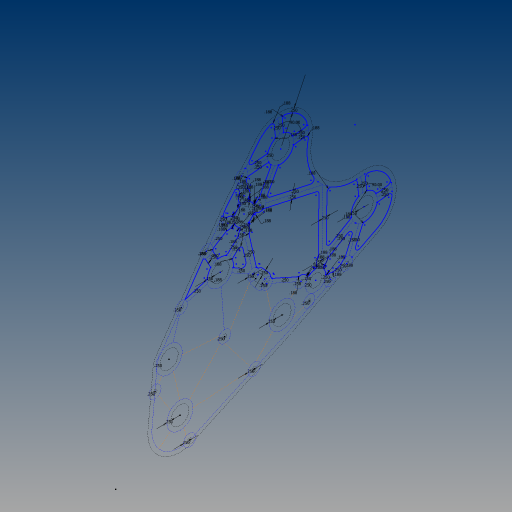
# Autodesk Inventor part: SHOT_1_001_ShooterPlate
Saved by Autodesk Inventor 2024.3 (Build 283343000, 343)
## iProperties
Created: 2024-08-07
Part Number: SHOT_1_001_ShooterPlate
Material: Aluminum 6061
Document SubType Name: Modeling
Designer: Kenji
Density: 2.7 g/cm^3
Appearance: Aluminum - Flat
Mass: 320.131 g
Surface Area: 825.953 cm^2
Volume: 118.567 cm^3
Author: Kenji
Autodesk Inventor part; units mm, degrees
ref_plane "YZ Plane" through (0, 0, 0) normal (1, 0, 0) x (0, 1, 0)
ref_plane "XZ Plane" through (0, 0, 0) normal (0, 1, 0) x (-1, 0, 0)
ref_plane "XY Plane" through (0, 0, 0) normal (0, 0, 1) x (1, 0, 0)
sketch "Sketch1" plane through (0, 0, 0) normal (1, 0, 0) x (0, 1, 0)
  line L0 (0, 0) -> (355.6, 0) construction
  line L1 (0, -355.6) -> (0, 0) construction
  line L2 (0, -292.1) -> (279.4, -292.1) construction
  circle A0 centre (336.7111, -261.0807) radius 50.8 construction
  circle A1 centre (191.0749, -393.5194) radius 50.8 construction
  circle A2 centre (263.893, -327.3) radius 50.8 construction
  circle A3 centre (191.0749, -393.5194) radius 47.625 construction
  circle A4 centre (336.7111, -261.0807) radius 47.625 construction
  line L3 (336.7111, -261.0807) -> (191.0749, -393.5194) construction
  circle A5 centre (336.7111, -261.0807) radius 14.2875
  circle A6 centre (191.0749, -393.5194) radius 14.2875
  circle A7 centre (215.3861, -165.4189) radius 25.4 construction
  circle A8 centre (107.6199, -263.4194) radius 25.4 construction
  circle A9 centre (107.6199, -263.4194) radius 22.225 construction
  circle A10 centre (215.3861, -165.4189) radius 22.225 construction
  circle A11 centre (215.3861, -165.4189) radius 14.2875
  circle A12 centre (107.6199, -263.4194) radius 14.2875
  line L4 (301.4765, -293.1223) -> (198.9433, -180.3717) construction
  line L5 (226.3095, -361.4778) -> (123.7762, -248.7272) construction
  circle A13 centre (161.3597, -214.5495) radius 50.8 construction
  line L6 (215.3861, -165.4189) -> (107.6199, -263.4194) construction
  circle A14 centre (50.8, -101.6) radius 50.8 construction
  circle A15 centre (25.4, -170.0653) radius 25.4 construction
  circle A16 centre (25.4, -170.0653) radius 22.225 construction
  circle A17 centre (25.4, -170.0653) radius 14.2875 construction
  circle A18 centre (136.3874, -84.4507) radius 25.4 construction
  circle A19 centre (136.3874, -84.4507) radius 22.225 construction
  circle A20 centre (136.3874, -84.4507) radius 14.2875
  circle A21 centre (50.8, -101.6) radius 14.2875
  circle A22 centre (41.2055, -25.7462) radius 25.4 construction
  circle A23 centre (41.2055, -25.7462) radius 22.225 construction
  circle A24 centre (41.2055, -25.7462) radius 14.2875 construction
  circle A25 centre (-111.1945, -98.7712) radius 50.8 construction
  circle A26 centre (41.2055, -98.7712) radius 50.8 construction
  line L7 (-111.1945, -47.9712) -> (41.2055, -47.9712) construction
  line L8 (-111.1945, -149.5712) -> (41.2055, -149.5712) construction
  circle A27 centre (276.2209, -203.0571) radius 30 construction
  circle A28 centre (276.2209, -203.0571) radius 25.4 construction
  circle A29 centre (301.6209, -203.0571) radius 2.794
  circle A30 centre (294.1814, -185.0966) radius 2.794
  circle A31 centre (276.2209, -177.6571) radius 2.794
  circle A32 centre (258.2604, -185.0966) radius 2.794
  circle A33 centre (250.8209, -203.0571) radius 2.794
  circle A34 centre (258.2604, -221.0177) radius 2.794
  circle A35 centre (276.2209, -228.4571) radius 2.794
  circle A36 centre (294.1814, -221.0177) radius 2.794
  circle A37 centre (276.2209, -203.0571) radius 9.652
  line L9 (250.7089, -187.273) -> (236.9862, -178.7828) construction
  circle A38 centre (276.2209, -203.0571) radius 9.5504 construction
  circle A39 centre (336.7111, -261.0807) radius 9.5504 construction
  circle A40 centre (336.7111, -261.0807) radius 14.3256 construction
  circle A41 centre (215.3861, -165.4189) radius 14.3256 construction
  circle A42 centre (136.3874, -84.4507) radius 14.3256 construction
  circle A43 centre (215.3861, -165.4189) radius 14.3256 construction
  circle A44 centre (123.5241, -172.549) radius 6.35 construction
  circle A45 centre (123.5241, -172.549) radius 3.2512
  line L10 (122.4294, -178.8039) -> (111.9989, -238.3998) construction
  arc A46 (325.875, -310.7115) -> (241.5089, -387.4324) centre (310.9542, -379.0508) ccw
  arc A47 (325.875, -310.7115) -> (368.3984, -221.3748) centre (336.7111, -261.0807) ccw
  arc A48 (145.82, -416.5983) -> (241.5089, -387.4324) centre (191.0749, -393.5194) ccw
  line L11 (138.8602, -59.1713) -> (55.7455, -51.0413)
  arc A49 (150.8617, -63.5783) -> (138.8602, -59.1713) centre (136.3874, -84.4507) ccw
  arc A50 (55.7455, -51.0413) -> (4.5541, -122.6227) centre (50.8, -101.6) ccw
  circle A51 centre (197.6195, -103.7307) radius 6.35 construction
  circle A52 centre (197.6195, -103.7307) radius 3.2512
  line L12 (161.503, -214.4192) -> (263.893, -327.3) construction
  circle A53 centre (128.5073, -316.6157) radius 30 construction
  circle A54 centre (128.5073, -316.6157) radius 25.4 construction
  circle A55 centre (152.1501, -307.3324) radius 2.794 construction
  line L13 (191.5627, -101.8236) -> (160.6148, -92.0791) construction
  line L14 (199.3769, -109.8327) -> (208.3565, -141.0111) construction
  line L15 (116.9032, -287.0622) -> (117.5428, -288.6911) construction
  circle A56 centre (128.5073, -316.6157) radius 22.86 construction
  circle A57 centre (107.6199, -263.4194) radius 34.29 construction
  circle A58 centre (138.661, -293.3334) radius 2.794
  circle A59 centre (119.224, -292.9729) radius 2.794 construction
  circle A60 centre (105.2251, -306.462) radius 2.794
  circle A61 centre (104.8646, -325.899) radius 2.794 construction
  circle A62 centre (118.3537, -339.8979) radius 2.794
  circle A63 centre (137.7907, -340.2584) radius 2.794 construction
  circle A64 centre (151.7896, -326.7693) radius 2.794
  line L16 (176.8412, -219.7225) -> (165.2897, -230.2004)
  line L17 (165.1271, -233.5371) -> (168.779, -237.5632)
  line L18 (172.1157, -237.7258) -> (183.6672, -227.2479)
  line L19 (183.8298, -223.9112) -> (180.1779, -219.8851)
  arc A65 (183.6672, -227.2479) -> (183.8298, -223.9112) centre (182.0802, -225.4982) ccw
  arc A66 (180.1779, -219.8851) -> (176.8412, -219.7225) centre (178.4283, -221.4722) ccw
  arc A67 (168.779, -237.5632) -> (172.1157, -237.7258) centre (170.5287, -235.9761) ccw
  arc A68 (165.2897, -230.2004) -> (165.1271, -233.5371) centre (166.8768, -231.9501) ccw
  line L20 (186.1428, -218.1439) -> (162.8049, -239.3128) construction
  circle A69 centre (186.1428, -218.1439) radius 2.3876
  circle A70 centre (162.8049, -239.3128) radius 2.3812
  circle A71 centre (128.5073, -316.6157) radius 9.5504
  circle A72 centre (276.2209, -203.0571) radius 30.48 construction
  circle A73 centre (336.7111, -261.0807) radius 41.91 construction
  circle A74 centre (276.2209, -203.0571) radius 41.91 construction
  circle A75 centre (128.5073, -316.6157) radius 19.1008 construction
  circle A76 centre (215.3861, -165.4189) radius 19.1008 construction
  circle A77 centre (136.3874, -84.4507) radius 19.1008 construction
  circle A78 centre (276.2209, -203.0571) radius 19.1008 construction
  circle A79 centre (191.0749, -393.5194) radius 19.1008 construction
  line L21 (4.5541, -122.6227) -> (75.2478, -278.1353)
  line L22 (75.9415, -279.5746) -> (145.82, -416.5983)
  arc A80 (75.2478, -278.1353) -> (75.9415, -279.5746) centre (107.6199, -263.4194) ccw
  circle A81 centre (276.2209, -203.0571) radius 43.18 construction
  line L23 (303.1551, -169.3072) -> (368.3984, -221.3748)
  line L24 (150.8617, -63.5783) -> (300.8271, -167.5741)
  arc A82 (303.1551, -169.3072) -> (300.8271, -167.5741) centre (276.2209, -203.0571) ccw
  circle A83 centre (107.6199, -263.4194) radius 35.56 construction
  circle A84 centre (126.9785, -365.675) radius 6.35 construction
  circle A85 centre (126.9785, -365.675) radius 3.2512
  circle A86 centre (330.5575, -199.3) radius 6.35 construction
  circle A87 centre (330.5575, -199.3) radius 3.2512
  circle A88 centre (255.1053, -143.5951) radius 6.35
  circle A89 centre (255.1053, -143.5951) radius 3.2512
  circle A90 centre (103.0707, -62.0508) radius 6.35 construction
  circle A91 centre (103.0707, -62.0508) radius 3.2512
  circle A92 centre (9.0853, -116.952) radius 6.35 construction
  circle A93 centre (9.0853, -116.952) radius 3.2512
  line L25 (37.3917, -106.5346) -> (15.0445, -114.7588) construction
  line L26 (10.9498, -123.0221) -> (17.9418, -145.7849) construction
  line L27 (108.3404, -65.5938) -> (115.3086, -70.2787) construction
  line L28 (98.0069, -65.8823) -> (91.3109, -70.9486) construction
  line L29 (257.2302, -149.579) -> (261.7713, -162.3666) construction
  line L30 (249.54, -146.6529) -> (237.6471, -153.1876) construction
  line L31 (331.1869, -205.6187) -> (331.6761, -210.5308) construction
  line L32 (324.2226, -199.738) -> (319.298, -200.0785) construction
  line L33 (127.1763, -359.3281) -> (127.5729, -346.6011) construction
  line L34 (132.8027, -368.2051) -> (144.4815, -373.2786) construction
  line L35 (38.6307, -191.7472) -> (52.2676, -214.0948) construction
  line L36 (80.4395, -240.4904) -> (60.4289, -223.6098) construction
  circle A94 centre (55.5753, -219.5153) radius 6.35 construction
  circle A95 centre (55.5753, -219.5153) radius 3.2512
  point P0 (33.8339, -53.7169)
  point P1 (178.5909, -218.1355)
  point P2 (163.5401, -231.7874)
  point P3 (170.3661, -239.3128)
  point P4 (171.0655, -224.9615)
  point P5 (182.0039, -221.8982)
  point P6 (182.0039, -221.8982)
  dimension "d44" = 101.6
  dimension "d60" = 28.575
  dimension "d81" = 60
  dimension "d82" = 50.8
  dimension "d102" = 12.7
  dimension "d269" = 50.8
  dimension "d13" = 355.6
  dimension "d14" = 355.6
  dimension "d15" = 292.1
  dimension "d29" = 101.6
  dimension "d31" = 3.175
  dimension "d36" = 28.575
  dimension "d38" = 50.8
  dimension "d39" = 3.175
  dimension "d41" = 28.575
  dimension "d42" = 152.4
  dimension "d43" = 152.4
  dimension "d46" = 279.4
  dimension "d47" = 101.6
  dimension "d50" = 101.6
  dimension "d51" = 145.6628
  dimension "d61" = 113.1223
  dimension "d77" = 101.6
  dimension "d78" = 101.6
  dimension "d79" = 152.4
  dimension "d80" = 41.2055
  dimension "d83" = 5.588
  dimension "d86" = 360
  dimension "d88" = 19.304
  dimension "d91" = 19.1008
  dimension "d92" = 19.1008
  dimension "d93" = 28.6512
  dimension "d94" = 28.6512
  dimension "d95" = 28.6512
  dimension "d96" = 28.6512
  dimension "d103" = 6.5024
  dimension "d108" = 12.7
  dimension "d109" = 6.5024
  dimension "d114" = 101.6
  dimension "d116" = 87.2886
  dimension "d117" = 158.0611
  dimension "d119" = 323.8734
  dimension "d121" = 42.21
  dimension "d268" = 60
  dimension "d270" = 5.588
  dimension "d279" = 45.72
  dimension "d280" = 68.58
  dimension "d283" = 360
  dimension "d285" = 20.32
  dimension "d286" = 10.16
  dimension "d287" = 10.16
  dimension "d288" = 2.3622
  dimension "d289" = 2.3622
  dimension "d291" = 5.08
  dimension "d292" = 4.7752
  dimension "d293" = 4.7625
  dimension "d294" = 5.6005
  dimension "d295" = 5.588
  dimension "d296" = 19.1008
  dimension "d297" = 60.96
  dimension "d300" = 83.82
  dimension "d301" = 83.82
  dimension "d302" = 38.2016
  dimension "d303" = 38.2016
  dimension "d304" = 38.2016
  dimension "d305" = 38.2016
  dimension "d306" = 38.2016
  dimension "d309" = 1.27
  dimension "d312" = 1.27
  dimension "d314" = 208.6282
  constraints: 89 centre point, 74 end point, 71 point on circle, 46 point on line, 46 tangent, 38 coincident, 18 equal radius, 7 equal length, 6 concentric, 6 midpoint, 5 perpendicular, 3 horizontal, 2 horizontal alignment, 2 parallel, 1 vertical alignment, 60 other
  measures "d13" distance of L1.start L0.start
  measures "d14" distance of L0.start L0.end
  measures "d15" distance between parallel lines of L0 L2
  measures "d29" diameter of A1
  measures "d31" radial gap between concentric circles of A1 A3
  measures "d36" diameter of A5
  measures "d38" diameter of A8
  measures "d39" radial gap between concentric circles of A8 A9
  measures "d41" diameter of A12
  measures "d42" distance of L4.start L4.end
  measures "d43" distance of L5.start L5.end
  measures "d46" distance of L2.start L2.end
  measures "d47" diameter of A14
  measures "d50" distance from line of L0 A14.centre
  measures "d51" distance of L6.start L6.end
  measures "d61" distance of A19.centre A7.centre
  measures "d77" diameter of A25
  measures "d78" diameter of A26
  measures "d79" distance of L8.start L8.end
  measures "d80" distance from line of L1 A22.centre
  measures "d83" diameter of A29
  measures "d88" diameter of A37
  measures "d91" diameter of A38
  measures "d92" diameter of A39
  measures "d93" diameter of A40
  measures "d94" diameter of A41
  measures "d95" diameter of A42
  measures "d96" diameter of A43
  measures "d103" diameter of A45
  measures "d108" diameter of A51
  measures "d109" diameter of A52
  measures "d114" distance of point (123.524, -172.549) A14.centre
  measures "d116" distance of A14.centre A19.centre
  measures "d117" distance of A14.centre L12.start
  measures "d119" distance of A14.centre L3.end
  measures "d121" angle of L1 L12
  measures "d268" diameter of A53
  measures "d270" diameter of A55
  measures "d279" diameter of A56
  measures "d280" diameter of A57
  measures "d285" distance of point (178.591, -218.135) point (163.54, -231.787)
  measures "d286" distance of point (163.54, -231.787) point (170.366, -239.313)
  measures "d287" distance of point (178.591, -218.135) point (171.065, -224.961)
  measures "d288" radius of A65
  measures "d289" radius of A67
  measures "d291" distance between parallel lines of L16 L20
  measures "d292" diameter of A69
  measures "d293" diameter of A70
  measures "d294" distance from line of L17 L20.end
  measures "d295" distance from line of L19 A69.centre
  measures "d296" diameter of A71
  measures "d297" diameter of A72
  measures "d300" diameter of A73
  measures "d301" diameter of A74
  measures "d302" diameter of A75
  measures "d303" diameter of A76
  measures "d304" diameter of A77
  measures "d305" diameter of A78
  measures "d306" diameter of A79
  measures "d309" radial gap between concentric circles of A74 A81
  measures "d312" radial gap between concentric circles of A57 A83
  measures "d314" distance of L3.end point (276.221, -203.057)
extrude "Extrusion6" add sketch "Sketch1" along normal blind 4.7625 contours A30 | A32 | A34 | A36 | A88 | A46 A48 L22 A80 L21 A50 L11 A49 L24 A82 L23 A47 | A85 | A87 | A89 | A91 | A93 | A95
extrude "Extrusion7" cut sketch "Sketch1" along normal blind 25.4 contours A85 | A87 | A89 | A91 | A93 | A95
sketch "Sketch5" plane through (4.7625, 0, 0) normal (1, 0, 0) x (0, 0, -1)
  circle A0 centre (62.0508, 103.0707) radius 3.2512 construction
  circle A1 centre (365.675, 126.9785) radius 3.2512 construction
  circle A2 centre (116.952, 9.0853) radius 3.2512 construction
  circle A3 centre (143.5951, 255.1053) radius 3.2512 construction
  circle A4 centre (199.3, 330.5575) radius 3.2512 construction
  circle A5 centre (219.5153, 55.5753) radius 3.2512 construction
  line L0 (167.5741, 300.8271) -> (63.5783, 150.8617) construction
  arc A6 (63.5783, 150.8617) -> (59.1713, 138.8602) centre (84.4507, 136.3874) ccw construction
  line L1 (59.1713, 138.8602) -> (51.0413, 55.7455) construction
  arc A7 (51.0413, 55.7455) -> (122.6227, 4.5541) centre (101.6, 50.8) ccw construction
  line L2 (122.6227, 4.5541) -> (278.1353, 75.2478) construction
  arc A8 (278.1353, 75.2478) -> (279.5746, 75.9415) centre (263.4194, 107.6199) ccw construction
  line L3 (279.5746, 75.9415) -> (416.5983, 145.82) construction
  arc A9 (416.5983, 145.82) -> (387.4324, 241.5089) centre (393.5194, 191.0749) ccw construction
  arc A10 (310.7115, 325.875) -> (387.4324, 241.5089) centre (379.0508, 310.9542) ccw construction
  arc A11 (310.7115, 325.875) -> (221.3748, 368.3984) centre (261.0807, 336.7111) ccw construction
  line L4 (221.3748, 368.3984) -> (169.3072, 303.1551) construction
  arc A12 (169.3072, 303.1551) -> (167.5741, 300.8271) centre (203.0571, 276.2209) ccw construction
  circle A13 centre (326.7693, 151.7896) radius 2.794 construction
  circle A14 centre (172.549, 123.5241) radius 3.2512 construction
  circle A15 centre (203.0571, 276.2209) radius 9.652 construction
  circle A16 centre (228.4571, 276.2209) radius 2.794 construction
  circle A17 centre (203.0571, 250.8209) radius 2.794 construction
  circle A18 centre (177.6571, 276.2209) radius 2.794 construction
  circle A19 centre (84.4507, 136.3874) radius 14.2875 construction
  circle A20 centre (263.4194, 107.6199) radius 14.2875 construction
  circle A21 centre (316.6157, 128.5073) radius 9.5504 construction
  circle A22 centre (239.3128, 162.8049) radius 2.3812 construction
  circle A23 centre (218.1439, 186.1428) radius 2.3876 construction
  arc A24 (219.8851, 180.1779) -> (219.7225, 176.8412) centre (221.4722, 178.4283) ccw construction
  line L5 (219.8851, 180.1779) -> (223.9112, 183.8298) construction
  arc A25 (227.2479, 183.6672) -> (223.9112, 183.8298) centre (225.4982, 182.0802) ccw construction
  line L6 (227.2479, 183.6672) -> (237.7258, 172.1157) construction
  arc A26 (237.5632, 168.779) -> (237.7258, 172.1157) centre (235.9761, 170.5287) ccw construction
  line L7 (237.5632, 168.779) -> (233.5371, 165.1271) construction
  arc A27 (230.2004, 165.2897) -> (233.5371, 165.1271) centre (231.9501, 166.8768) ccw construction
  line L8 (230.2004, 165.2897) -> (219.7225, 176.8412) construction
  circle A28 centre (339.8979, 118.3537) radius 2.794 construction
  circle A29 centre (306.462, 105.2251) radius 2.794 construction
  circle A30 centre (293.3334, 138.661) radius 2.794 construction
  circle A31 centre (103.7307, 197.6195) radius 3.2512 construction
  circle A32 centre (203.0571, 301.6209) radius 2.794 construction
  circle A33 centre (101.6, 50.8) radius 14.2875 construction
  circle A34 centre (165.4189, 215.3861) radius 14.2875 construction
  circle A35 centre (393.5194, 191.0749) radius 14.2875 construction
  circle A36 centre (261.0807, 336.7111) radius 14.2875 construction
  arc A37 (304.5076, 327.2295) -> (226.3381, 364.4375) centre (261.0807, 336.7111) ccw construction
  arc A38 (304.5076, 327.2295) -> (388.1933, 235.2047) centre (379.0508, 310.9542) ccw construction
  arc A39 (413.7134, 151.4769) -> (388.1933, 235.2047) centre (393.5194, 191.0749) ccw construction
  line L9 (413.7134, 151.4769) -> (276.6898, 81.5983) construction
  arc A40 (275.5075, 81.0285) -> (276.6898, 81.5983) centre (263.4194, 107.6199) ccw construction
  line L10 (275.5075, 81.0285) -> (119.9949, 10.3348) construction
  arc A41 (57.3611, 55.1273) -> (119.9949, 10.3348) centre (101.6, 50.8) ccw construction
  line L11 (57.3611, 55.1273) -> (65.4912, 138.242) construction
  arc A42 (68.7964, 147.2431) -> (65.4912, 138.242) centre (84.4507, 136.3874) ccw construction
  line L12 (68.7964, 147.2431) -> (172.7922, 297.2086) construction
  arc A43 (174.2704, 299.1942) -> (172.7922, 297.2086) centre (203.0571, 276.2209) ccw construction
  line L13 (174.2704, 299.1942) -> (226.3381, 364.4375) construction
  circle A44 centre (261.0807, 336.7111) radius 20.6375 construction
  circle A45 centre (199.3, 330.5575) radius 9.6012 construction
  circle A46 centre (203.0571, 301.6209) radius 9.144 construction
  circle A47 centre (228.4571, 276.2209) radius 9.144 construction
  circle A48 centre (203.0571, 276.2209) radius 16.002 construction
  circle A49 centre (177.6571, 276.2209) radius 9.144 construction
  circle A50 centre (203.0571, 250.8209) radius 9.144 construction
  circle A51 centre (143.5951, 255.1053) radius 9.6012 construction
  circle A52 centre (165.4189, 215.3861) radius 20.6375 construction
  circle A53 centre (103.7307, 197.6195) radius 9.6012 construction
  circle A54 centre (84.4507, 136.3874) radius 20.6375 construction
  circle A55 centre (62.0508, 103.0707) radius 9.6012 construction
  circle A56 centre (172.549, 123.5241) radius 9.6012 construction
  circle A57 centre (101.6, 50.8) radius 20.6375 construction
  circle A58 centre (116.952, 9.0853) radius 9.6012 construction
  circle A59 centre (219.5153, 55.5753) radius 9.6012 construction
  circle A60 centre (263.4194, 107.6199) radius 20.6375 construction
  circle A61 centre (218.1439, 186.1428) radius 8.7376 construction
  line L14 (242.4292, 176.382) -> (231.9513, 187.9335) construction
  arc A62 (231.9513, 187.9335) -> (219.6449, 188.5332) centre (225.4982, 182.0802) ccw construction
  line L15 (219.6449, 188.5332) -> (215.6189, 184.8813) construction
  arc A63 (215.6189, 184.8813) -> (215.0191, 172.575) centre (221.4722, 178.4283) ccw construction
  line L16 (215.0191, 172.575) -> (225.497, 161.0235) construction
  arc A64 (225.497, 161.0235) -> (237.8033, 160.4238) centre (231.9501, 166.8768) ccw construction
  line L17 (237.8033, 160.4238) -> (241.8294, 164.0757) construction
  arc A65 (241.8294, 164.0757) -> (242.4292, 176.382) centre (235.9761, 170.5287) ccw construction
  circle A66 centre (239.3128, 162.8049) radius 8.7312 construction
  circle A67 centre (393.5194, 191.0749) radius 20.6375 construction
  circle A68 centre (326.7693, 151.7896) radius 9.144 construction
  circle A69 centre (293.3334, 138.661) radius 9.144 construction
  circle A70 centre (316.6157, 128.5073) radius 15.9004 construction
  circle A71 centre (365.675, 126.9785) radius 9.6012 construction
  circle A72 centre (339.8979, 118.3537) radius 9.144 construction
  circle A73 centre (306.462, 105.2251) radius 9.144 construction
  line L18 (240.5448, 334.6656) -> (208.8539, 331.5091) construction
  line L19 (259.0352, 357.247) -> (256.6751, 380.9422) construction
  line L20 (281.6165, 338.7565) -> (305.3118, 341.1167) construction
  line L21 (251.2843, 318.5469) -> (232.7977, 284.269) construction
  line L22 (200.5362, 321.0362) -> (201.8798, 310.6888) construction
  line L23 (170.1431, 281.4316) -> (164.544, 285.3144) construction
  line L24 (148.2185, 246.6906) -> (155.4809, 233.4731) construction
  line L25 (151.7555, 260.1641) -> (169.8853, 271.403) construction
  line L26 (205.0841, 241.9044) -> (215.844, 194.5723) construction
  line L27 (183.5074, 205.4507) -> (210.6081, 190.5652) construction
  line L28 (180.4451, 229.5325) -> (196.3994, 244.5529) construction
  line L29 (252.4974, 358.8173) -> (250.9874, 373.9773)
  line L30 (237.7157, 340.7653) -> (216.1032, 338.6126)
  line L31 (211.8976, 346.3429) -> (226.3381, 364.4375)
  arc A74 (244.449, 377.9323) -> (226.3381, 364.4375) centre (261.0807, 336.7111) ccw
  arc A75 (250.2514, 354.2791) -> (241.7218, 343.8623) centre (261.0807, 336.7111) ccw
  arc A76 (250.2514, 354.2791) -> (252.4974, 358.8173) centre (247.7457, 358.344) ccw
  arc A77 (237.7157, 340.7653) -> (241.7218, 343.8623) centre (237.2424, 345.5169) ccw
  arc A78 (211.8976, 346.3429) -> (216.1032, 338.6126) centre (215.6299, 343.3643) ccw
  arc A79 (250.9874, 373.9773) -> (244.449, 377.9323) centre (246.2357, 373.504) ccw
  line L32 (238.9744, 328.1278) -> (211.3352, 325.3748)
  line L33 (207.073, 320.0083) -> (208.2772, 310.7339)
  line L34 (244.646, 319.6154) -> (226.8389, 286.5977)
  arc A80 (206.5244, 324.2336) -> (207.0953, 324.9525) centre (199.3, 330.5575) ccw
  arc A81 (243.5127, 325.8818) -> (244.321, 324.6686) centre (261.0807, 336.7111) ccw
  line L35 (219.0591, 276.2209) -> (219.3131, 276.2209) construction
  line L36 (203.0571, 292.4769) -> (203.0571, 292.2229) construction
  line L37 (209.4071, 294.0954) -> (209.4071, 292.4021)
  line L38 (219.2384, 282.5709) -> (220.9317, 282.5709)
  arc A82 (209.9856, 295.6536) -> (209.5973, 308.0115) centre (203.0571, 301.6209) ccw
  arc A83 (217.1375, 283.824) -> (210.6603, 290.3012) centre (203.0571, 276.2209) ccw
  arc A84 (224.633, 284.5268) -> (222.4898, 283.1494) centre (228.4571, 276.2209) ccw
  arc A85 (211.3352, 325.3748) -> (207.073, 320.0083) centre (211.8085, 320.6231) ccw
  arc A86 (243.5127, 325.8818) -> (238.9744, 328.1278) centre (239.4477, 323.3761) ccw
  arc A87 (244.646, 319.6154) -> (244.321, 324.6686) centre (240.4431, 321.8822) ccw
  arc A88 (224.633, 284.5268) -> (226.8389, 286.5977) centre (222.636, 288.8644) ccw
  arc A89 (208.2772, 310.7339) -> (209.5973, 308.0115) centre (213.0127, 311.3488) ccw
  circle A90 centre (211.7947, 294.0954) radius 2.3876 construction
  circle A91 centre (220.9317, 284.9585) radius 2.3876 construction
  circle A92 centre (219.2384, 284.9585) radius 2.3876 construction
  circle A93 centre (211.7947, 292.4021) radius 2.3876 construction
  arc A94 (217.1375, 283.824) -> (219.2384, 282.5709) centre (219.2384, 284.9585) ccw
  arc A95 (220.9317, 282.5709) -> (222.4898, 283.1494) centre (220.9317, 284.9585) ccw
  arc A96 (209.4071, 292.4021) -> (210.6603, 290.3012) centre (211.7947, 292.4021) ccw
  arc A97 (209.9856, 295.6536) -> (209.4071, 294.0954) centre (211.7947, 294.0954) ccw
  line L39 (328.2576, 254.0189) -> (237.3829, 274.2352) construction
  line L40 (328.2576, 254.0189) -> (326.9024, 160.9326) construction
  line L41 (255.824, 313.5869) -> (241.0284, 286.1531)
  line L42 (244.1944, 279.2252) -> (308.259, 264.9731)
  line L43 (284.4456, 332.6569) -> (299.6056, 334.1669)
  arc A98 (260.2249, 316.0913) -> (280.4395, 329.5599) centre (261.0807, 336.7111) ccw
  arc A99 (304.5076, 327.2295) -> (304.7726, 328.5371) centre (261.0807, 336.7111) ccw
  arc A100 (304.5076, 327.2295) -> (313.4045, 272.0681) centre (379.0508, 310.9542) ccw
  arc A101 (304.7726, 328.5371) -> (299.6056, 334.1669) centre (300.0789, 329.4152) ccw
  arc A102 (308.259, 264.9731) -> (313.4045, 272.0681) centre (309.296, 269.6344) ccw
  arc A103 (241.0284, 286.1531) -> (244.1944, 279.2252) centre (245.2313, 283.8864) ccw
  arc A104 (260.2249, 316.0913) -> (255.824, 313.5869) centre (260.0269, 311.3202) ccw
  arc A105 (284.4456, 332.6569) -> (280.4395, 329.5599) centre (284.9189, 327.9052) ccw
  line L44 (283.1869, 345.2944) -> (298.3468, 346.8044)
  line L45 (265.1348, 360.076) -> (263.6248, 375.236)
  arc A106 (302.3019, 353.3428) -> (269.2547, 380.403) centre (261.0807, 336.7111) ccw
  arc A107 (278.6486, 347.5403) -> (268.2318, 356.07) centre (261.0807, 336.7111) ccw
  arc A108 (269.2547, 380.403) -> (263.6248, 375.236) centre (268.3765, 375.7093) ccw
  arc A109 (298.3468, 346.8044) -> (302.3019, 353.3428) centre (297.8735, 351.556) ccw
  arc A110 (278.6486, 347.5403) -> (283.1869, 345.2944) centre (282.7136, 350.046) ccw
  arc A111 (265.1348, 360.076) -> (268.2318, 356.07) centre (269.8865, 360.5493) ccw
  line L46 (235.2436, 268.2059) -> (318.0387, 249.787)
  line L47 (321.7764, 245.0563) -> (320.5418, 160.2462)
  line L48 (211.1035, 244.0716) -> (222.1565, 195.4498)
  line L49 (203.0571, 260.2189) -> (203.0571, 259.9649) construction
  line L50 (209.4071, 260.0397) -> (209.4071, 258.3463)
  line L51 (247.2842, 159.2422) -> (284.9853, 142.3921) construction
  line L52 (248.8959, 165.4772) -> (288.2875, 147.8716)
  line L53 (301.715, 135.0057) -> (302.041, 134.8635) construction
  line L54 (323.114, 143.408) -> (322.9719, 143.082) construction
  line L55 (302.7698, 141.4733) -> (304.4279, 140.7502)
  line L56 (317.6048, 146.6604) -> (317.2174, 145.7719)
  arc A112 (301.5729, 142.6264) -> (291.2986, 147.5757) centre (293.3334, 138.661) ccw
  arc A113 (319.5416, 157.3907) -> (317.8734, 149.6741) centre (326.7693, 151.7896) ccw
  arc A114 (315.236, 144.3478) -> (306.8489, 141.0546) centre (316.6157, 128.5073) ccw
  line L57 (219.2384, 269.8709) -> (220.9317, 269.8709)
  arc A115 (222.4898, 269.2924) -> (232.2342, 267.8934) centre (228.4571, 276.2209) ccw
  arc A116 (210.6603, 262.1405) -> (217.1375, 268.6177) centre (203.0571, 276.2209) ccw
  arc A117 (211.402, 247.0824) -> (209.9856, 256.7882) centre (203.0571, 250.8209) ccw
  arc A118 (235.2436, 268.2059) -> (232.2342, 267.8934) centre (234.2067, 263.5446) ccw
  arc A119 (321.7764, 245.0563) -> (318.0387, 249.787) centre (317.0017, 245.1258) ccw
  arc A120 (319.5416, 157.3907) -> (320.5418, 160.2462) centre (315.7671, 160.3157) ccw
  arc A121 (317.6048, 146.6604) -> (317.8734, 149.6741) centre (313.2278, 148.5693) ccw
  arc A122 (224.5561, 192.0782) -> (223.7494, 192.8453) centre (218.1439, 186.1428) ccw
  arc A123 (231.9513, 187.9335) -> (227.1533, 190.6337) centre (225.4982, 182.0802) ccw
  arc A124 (246.7674, 167.3507) -> (245.8371, 168.6073) centre (239.3128, 162.8049) ccw
  arc A125 (244.6507, 171.3375) -> (242.4292, 176.382) centre (235.9761, 170.5287) ccw
  line L58 (231.9513, 187.9335) -> (242.4292, 176.382)
  arc A126 (211.402, 247.0824) -> (211.1035, 244.0716) centre (215.7599, 245.1301) ccw
  arc A127 (222.1565, 195.4498) -> (223.7494, 192.8453) centre (226.8129, 196.5083) ccw
  arc A128 (224.5561, 192.0782) -> (227.1533, 190.6337) centre (228.0605, 195.3219) ccw
  arc A129 (244.6507, 171.3375) -> (245.8371, 168.6073) centre (249.4053, 171.7808) ccw
  arc A130 (246.7674, 167.3507) -> (248.8959, 165.4772) centre (250.8444, 169.8368) ccw
  arc A131 (288.2875, 147.8716) -> (291.2986, 147.5757) centre (290.2359, 152.2312) ccw
  circle A132 centre (211.7947, 258.3463) radius 2.3876 construction
  circle A133 centre (211.7947, 260.0397) radius 2.3876 construction
  circle A134 centre (220.9317, 267.4833) radius 2.3876 construction
  circle A135 centre (219.2384, 267.4833) radius 2.3876 construction
  arc A136 (219.2384, 269.8709) -> (217.1375, 268.6177) centre (219.2384, 267.4833) ccw
  arc A137 (222.4898, 269.2924) -> (220.9317, 269.8709) centre (220.9317, 267.4833) ccw
  arc A138 (210.6603, 262.1405) -> (209.4071, 260.0397) centre (211.7947, 260.0397) ccw
  arc A139 (209.4071, 258.3463) -> (209.9856, 256.7882) centre (211.7947, 258.3463) ccw
  circle A140 centre (315.0288, 146.7264) radius 2.3876 construction
  circle A141 centre (303.7243, 143.6618) radius 2.3876 construction
  circle A142 centre (305.3824, 142.9387) radius 2.3876 construction
  arc A143 (315.236, 144.3478) -> (317.2174, 145.7719) centre (315.0288, 146.7264) ccw
  arc A144 (301.5729, 142.6264) -> (302.7698, 141.4733) centre (303.7243, 143.6618) ccw
  arc A145 (304.4279, 140.7502) -> (306.8489, 141.0546) centre (305.3824, 142.9387) ccw
  line L59 (385.2966, 172.1463) -> (369.5005, 135.7847) construction
  line L60 (375.7337, 180.6072) -> (334.6498, 156.4276) construction
  line L61 (391.0466, 211.5637) -> (388.1933, 235.2047) construction
  line L62 (414.0082, 193.5478) -> (437.6492, 196.4011) construction
  line L63 (333.4067, 171.4846) -> (334.4104, 240.4277)
  line L64 (370.6077, 184.9585) -> (340.6035, 167.2997)
  line L65 (384.4774, 212.9975) -> (382.3693, 230.4644)
  arc A146 (382.3265, 208.4134) -> (372.946, 189.4499) centre (393.5194, 191.0749) ccw
  arc A147 (341.5331, 244.5162) -> (377.7123, 234.6667) centre (379.0508, 310.9542) ccw
  arc A148 (341.5331, 244.5162) -> (334.4104, 240.4277) centre (339.1851, 240.3582) ccw
  arc A149 (382.3693, 230.4644) -> (377.7123, 234.6667) centre (377.6285, 229.8922) ccw
  arc A150 (382.3265, 208.4134) -> (384.4774, 212.9975) centre (379.7366, 212.4253) ccw
  arc A151 (370.6077, 184.9585) -> (372.946, 189.4499) centre (368.1856, 189.0739) ccw
  arc A152 (333.4067, 171.4846) -> (340.6035, 167.2997) centre (338.1814, 171.4151) ccw
  line L66 (367.2672, 168.2562) -> (337.1993, 150.5599)
  line L67 (374.069, 162.2382) -> (363.4789, 137.8602)
  line L68 (348.5694, 121.2551) -> (356.57, 123.932) construction
  line L69 (345.8158, 127.0298) -> (355.0252, 130.1112)
  arc A153 (361.2833, 135.5164) -> (357.5507, 132.0949) centre (365.675, 126.9785) ccw
  arc A154 (355.0252, 130.1112) -> (357.5507, 132.0949) centre (353.51, 134.6396) ccw
  arc A155 (361.2833, 135.5164) -> (363.4789, 137.8602) centre (359.0991, 139.7628) ccw
  arc A156 (374.069, 162.2382) -> (367.2672, 168.2562) centre (369.6893, 164.1408) ccw
  line L70 (397.0859, 214.5193) -> (395.2604, 229.6445)
  line L71 (415.442, 200.1169) -> (430.5672, 201.9424)
  line L72 (416.9638, 187.5084) -> (432.089, 189.3339)
  line L73 (390.24, 167.5887) -> (379.8681, 143.7131)
  line L74 (386.4173, 137.5565) -> (413.7134, 151.4769)
  arc A157 (410.858, 202.2678) -> (400.2657, 210.5786) centre (393.5194, 191.0749) ccw
  arc A158 (434.3852, 208.5618) -> (400.7814, 234.9277) centre (393.5194, 191.0749) ccw
  arc A159 (413.7134, 151.4769) -> (437.3722, 183.813) centre (393.5194, 191.0749) ccw
  arc A160 (394.413, 170.4568) -> (413.0231, 184.3286) centre (393.5194, 191.0749) ccw
  arc A161 (397.0859, 214.5193) -> (400.2657, 210.5786) centre (401.8267, 215.0914) ccw
  arc A162 (410.858, 202.2678) -> (415.442, 200.1169) centre (414.8698, 204.8577) ccw
  arc A163 (430.5672, 201.9424) -> (434.3852, 208.5618) centre (429.995, 206.6832) ccw
  arc A164 (400.7814, 234.9277) -> (395.2604, 229.6445) centre (400.0012, 230.2167) ccw
  arc A165 (416.9638, 187.5084) -> (413.0231, 184.3286) centre (417.536, 182.7676) ccw
  arc A166 (394.413, 170.4568) -> (390.24, 167.5887) centre (394.6197, 165.686) ccw
  arc A167 (379.8681, 143.7131) -> (386.4173, 137.5565) centre (384.2479, 141.8105) ccw
  arc A168 (437.3722, 183.813) -> (432.089, 189.3339) centre (432.6612, 184.5931) ccw
  line L75 (195.2416, 312.4978) -> (195.6829, 309.0987)
  line L76 (174.4018, 286.2058) -> (172.0866, 287.8113)
  line L77 (186.8011, 276.2209) -> (187.0551, 276.2209) construction
  line L78 (186.0222, 282.5709) -> (186.8759, 282.5709)
  line L79 (196.7071, 294.0954) -> (196.7071, 292.4021)
  arc A169 (195.1019, 306.1294) -> (196.1286, 295.6536) centre (203.0571, 301.6209) ccw
  arc A170 (193.3111, 323.0531) -> (193.9301, 322.5984) centre (199.3, 330.5575) ccw
  arc A171 (195.454, 290.3012) -> (188.9768, 283.824) centre (203.0571, 276.2209) ccw
  arc A172 (183.1524, 283.5294) -> (177.3062, 285.3581) centre (177.6571, 276.2209) ccw
  line L80 (170.8837, 294.4565) -> (172.7922, 297.2086)
  line L81 (174.2704, 299.1942) -> (186.7738, 314.8615)
  arc A173 (174.2704, 299.1942) -> (172.7922, 297.2086) centre (203.0571, 276.2209) ccw
  arc A174 (174.4018, 286.2058) -> (177.3062, 285.3581) centre (177.1229, 290.1298) ccw
  arc A175 (183.1524, 283.5294) -> (186.0222, 282.5709) centre (186.0222, 287.3461) ccw
  arc A176 (195.1019, 306.1294) -> (195.6829, 309.0987) centre (190.9475, 308.4838) ccw
  arc A177 (195.2416, 312.4978) -> (186.7738, 314.8615) centre (190.5061, 311.8829) ccw
  arc A178 (170.8837, 294.4565) -> (172.0866, 287.8113) centre (174.8077, 291.7353) ccw
  circle A179 centre (186.8759, 284.9585) radius 2.3876 construction
  arc A180 (186.8759, 282.5709) -> (188.9768, 283.824) centre (186.8759, 284.9585) ccw
  circle A181 centre (194.3195, 292.4021) radius 2.3876 construction
  circle A182 centre (194.3195, 294.0954) radius 2.3876 construction
  arc A183 (196.7071, 294.0954) -> (196.1286, 295.6536) centre (194.3195, 294.0954) ccw
  arc A184 (195.454, 290.3012) -> (196.7071, 292.4021) centre (194.3195, 292.4021) ccw
  line L82 (196.7071, 260.0397) -> (196.7071, 259.1859)
  line L83 (185.1826, 269.8709) -> (185.5094, 269.8709)
  arc A185 (189.5424, 267.6526) -> (195.454, 262.1405) centre (203.0571, 276.2209) ccw
  line L84 (155.9126, 255.2699) -> (173.8931, 266.4164)
  line L85 (154.2435, 248.9118) -> (159.9817, 238.4684)
  line L86 (177.7018, 235.6713) -> (192.6138, 249.7103)
  arc A186 (172.7356, 234.683) -> (164.402, 235.9985) centre (165.4189, 215.3861) ccw
  arc A187 (152.6282, 251.8517) -> (153.0616, 253.5026) centre (143.5951, 255.1053) ccw
  arc A188 (176.8373, 267.1137) -> (183.6244, 269.2924) centre (177.6571, 276.2209) ccw
  arc A189 (195.7486, 256.3162) -> (194.0462, 252.3753) centre (203.0571, 250.8209) ccw
  arc A190 (155.9126, 255.2699) -> (154.2435, 248.9118) centre (158.4286, 251.2113) ccw
  arc A191 (159.9817, 238.4684) -> (164.402, 235.9985) centre (164.1668, 240.7679) ccw
  arc A192 (172.7356, 234.683) -> (177.7018, 235.6713) centre (174.4285, 239.1481) ccw
  arc A193 (192.6138, 249.7103) -> (194.0462, 252.3753) centre (189.3405, 253.1871) ccw
  arc A194 (176.8373, 267.1137) -> (173.8931, 266.4164) centre (176.4091, 262.3577) ccw
  arc A195 (189.5424, 267.6526) -> (185.5094, 269.8709) centre (185.5094, 265.0957) ccw
  arc A196 (195.7486, 256.3162) -> (196.7071, 259.1859) centre (191.9319, 259.1859) ccw
  circle A197 centre (194.3195, 260.0397) radius 2.3876 construction
  circle A198 centre (185.1826, 267.4833) radius 2.3876 construction
  arc A199 (196.7071, 260.0397) -> (195.454, 262.1405) centre (194.3195, 260.0397) ccw
  arc A200 (185.1826, 269.8709) -> (183.6244, 269.2924) centre (185.1826, 267.4833) ccw
  line L87 (331.1904, 122.1511) -> (331.5163, 122.009) construction
  line L88 (335.1284, 127.3613) -> (335.5383, 127.1825)
  arc A201 (342.7902, 127.0282) -> (337.1978, 127.0899) centre (339.8979, 118.3537) ccw
  line L89 (329.246, 141.5836) -> (328.8585, 140.6951)
  arc A202 (331.2718, 143.8309) -> (335.2123, 148.2783) centre (326.7693, 151.7896) ccw
  arc A203 (332.3207, 130.9922) -> (329.1629, 138.2741) centre (316.6157, 128.5073) ccw
  arc A204 (342.7902, 127.0282) -> (345.8158, 127.0298) centre (344.3006, 131.5582) ccw
  arc A205 (337.1993, 150.5599) -> (335.2123, 148.2783) centre (339.6214, 146.4446) ccw
  arc A206 (331.2718, 143.8309) -> (329.246, 141.5836) centre (333.623, 139.6747) ccw
  arc A207 (332.3207, 130.9922) -> (335.1284, 127.3613) centre (337.0372, 131.7384) ccw
  circle A208 centre (336.4928, 129.3711) radius 2.3876 construction
  circle A209 centre (331.047, 139.7406) radius 2.3876 construction
  arc A210 (328.8585, 140.6951) -> (329.1629, 138.2741) centre (331.047, 139.7406) ccw
  arc A211 (335.5383, 127.1825) -> (337.1978, 127.0899) centre (336.4928, 129.3711) ccw
  line L90 (186.4073, 226.4244) -> (193.2473, 232.864)
  line L91 (201.177, 230.4457) -> (205.9543, 209.4304)
  line L92 (188.5021, 209.9521) -> (198.999, 204.1865)
  arc A212 (201.177, 230.4457) -> (193.2473, 232.864) centre (196.5206, 229.3871) ccw
  arc A213 (198.999, 204.1865) -> (205.9543, 209.4304) centre (201.2979, 208.3719) ccw
  arc A214 (186.0315, 214.3721) -> (185.1217, 221.5267) centre (165.4189, 215.3861) ccw
  arc A215 (186.4073, 226.4244) -> (185.1217, 221.5267) centre (189.6806, 222.9476) ccw
  arc A216 (186.0315, 214.3721) -> (188.5021, 209.9521) centre (190.801, 214.1375) ccw
  line L93 (145.5875, 209.6745) -> (112.9569, 200.2767) construction
  line L94 (167.016, 194.8105) -> (171.806, 133.0965) construction
  line L95 (100.8472, 188.4616) -> (90.6488, 156.0722) construction
  line L96 (72.9251, 119.2682) -> (67.8413, 111.1006) construction
  line L97 (104.627, 132.0487) -> (164.4098, 128.6168) construction
  line L98 (181.2176, 127.6519) -> (212.8239, 179.2115) construction
  line L99 (238.7786, 154.09) -> (246.3835, 119.2682) construction
  line L100 (248.8959, 92.958) -> (222.4898, 64.7041) construction
  line L101 (172.8037, 113.9263) -> (212.8239, 62.4606) construction
  line L102 (116.8506, 64.7041) -> (165.6161, 116.882) construction
  line L103 (101.6, 71.4375) -> (91.192, 116.882) construction
  line L104 (86.7938, 65.1765) -> (67.8413, 95.4121) construction
  line L105 (108.0861, 31.2083) -> (111.3646, 16.8933) construction
  line L106 (122.2375, 50.8) -> (209.9645, 56.5574) construction
  line L107 (86.7938, 36.4235) -> (67.9432, 21.7651) construction
  line L108 (286.2294, 132.9038) -> (277.0671, 123.1005) construction
  line L109 (279.0633, 94.1597) -> (298.0113, 101.7326) construction
  line L110 (141.4977, 245.736) -> (148.8512, 232.3527)
  line L111 (141.7059, 215.1647) -> (109.4568, 205.8768)
  line L112 (109.4568, 205.8768) -> (138.1238, 247.2155)
  arc A217 (138.1238, 247.2155) -> (141.4977, 245.736) centre (143.5951, 255.1053) ccw
  arc A218 (148.5657, 227.2972) -> (145.0885, 218.9327) centre (165.4189, 215.3861) ccw
  arc A219 (141.7059, 215.1647) -> (145.0885, 218.9327) centre (140.3843, 219.7534) ccw
  arc A220 (148.5657, 227.2972) -> (148.8512, 232.3527) centre (144.6661, 230.0532) ccw
  point P0 (0, 0)
  point P1 (217.6319, 186.7072)
  point P2 (252.8157, 355.6213)
  point P3 (250.4015, 379.8592)
  point P4 (240.9117, 341.0836)
  point P5 (205.8366, 337.59)
  point P6 (205.2889, 338.0619)
  point P7 (242.1704, 328.4461)
  point P8 (208.5071, 308.9633)
  point P9 (246.1706, 322.4423)
  point P10 (225.9914, 285.0261)
  point P11 (257.3486, 316.4138)
  point P12 (320.2776, 262.2994)
  point P13 (281.2496, 332.3386)
  point P14 (305.4875, 334.7527)
  point P15 (279.9909, 344.976)
  point P16 (304.2288, 347.3902)
  point P17 (265.4532, 356.8801)
  point P18 (263.039, 381.1179)
  point P19 (233.5007, 268.5936)
  point P20 (320.5158, 158.4609)
  point P21 (210.7077, 245.8126)
  point P22 (222.558, 193.6834)
  point P23 (247.375, 166.157)
  point P24 (289.9176, 147.143)
  point P25 (318.3186, 148.2971)
  point P26 (334.535, 248.9871)
  point P27 (373.3757, 186.5876)
  point P28 (384.8623, 209.8088)
  point P29 (381.8573, 234.7066)
  point P30 (379.8173, 175.6425)
  point P31 (335.6605, 149.6543)
  point P32 (379.8713, 175.5947)
  point P33 (362.7202, 136.1137)
  point P34 (344.1226, 126.4632)
  point P35 (356.8309, 130.7153)
  point P36 (344.1226, 126.4632)
  point P37 (335.6605, 149.6543)
  point P38 (397.4708, 211.3306)
  point P39 (394.5521, 235.5129)
  point P40 (412.2534, 199.7321)
  point P41 (436.4357, 202.6507)
  point P42 (413.7751, 187.1236)
  point P43 (437.9574, 190.0422)
  point P44 (391.5197, 170.5345)
  point P45 (374.5686, 131.514)
  point P46 (195.9128, 307.328)
  point P47 (175.869, 285.1883)
  point P48 (168.1626, 290.5325)
  point P49 (184.2367, 282.5709)
  point P50 (196.7071, 257.4004)
  point P51 (188.369, 269.8709)
  point P52 (175.4107, 267.3571)
  point P53 (161.5283, 235.6535)
  point P54 (175.3633, 233.4696)
  point P55 (193.9138, 250.9342)
  point P56 (329.9597, 143.2202)
  point P57 (332.5161, 128.5006)
  point P58 (184.0688, 224.2228)
  point P59 (185.687, 211.4984)
  point P60 (150.3978, 229.5378)
  point P61 (144.7922, 216.0536)
  dimension "d330" = 6.35
  dimension "d331" = 6.35
  dimension "d332" = 6.35
  dimension "d333" = 6.35
  dimension "d334" = 6.35
  dimension "d335" = 6.35
  dimension "d336" = 6.35
  dimension "d337" = 6.35
  dimension "d338" = 6.35
  dimension "d339" = 6.35
  dimension "d340" = 6.35
  dimension "d341" = 6.35
  dimension "d342" = 6.35
  dimension "d343" = 6.35
  dimension "d344" = 6.35
  dimension "d345" = 6.35
  dimension "d346" = 6.35
  dimension "d347" = 6.35
  dimension "d348" = 6.35
  dimension "d349" = 6.35
  dimension "d350" = 6.35
  dimension "d351" = 6.35
  dimension "d352" = 6.35
  dimension "d353" = 6.35
  dimension "d354" = 6.35
  dimension "d355" = 6.35
  dimension "d356" = 6.35
  dimension "d357" = 6.35
  dimension "d358" = 90
  dimension "d359" = 6.35
  dimension "d360" = 6.35
  dimension "d361" = 4.7752
  dimension "d362" = 4.7752
  dimension "d363" = 6.35
  dimension "d364" = 6.35
  dimension "d365" = 6.35
  dimension "d366" = 6.35
  dimension "d367" = 6.35
  dimension "d368" = 4.7752
  dimension "d369" = 4.7752
  dimension "d370" = 4.7752
  dimension "d371" = 4.7752
  dimension "d372" = 4.7752
  dimension "d373" = 4.7752
  dimension "d374" = 4.7752
  dimension "d375" = 6.35
  dimension "d376" = 6.35
  dimension "d377" = 6.35
  dimension "d378" = 4.7752
  dimension "d379" = 6.35
  dimension "d380" = 6.35
  dimension "d381" = 4.7752
  dimension "d382" = 6.35
  dimension "d383" = 6.35
  dimension "d384" = 6.35
  dimension "d385" = 6.35
  dimension "d386" = 6.35
  dimension "d387" = 6.35
  dimension "d388" = 6.35
  dimension "d389" = 4.7752
  dimension "d390" = 4.7752
  dimension "d391" = 4.7752
  dimension "d392" = 4.7752
  dimension "d393" = 4.7752
  constraints: 442 point on circle, 208 end point, 178 tangent, 171 centre point, 127 point on line, 44 parallel, 39 equal radius, 36 concentric, 4 collinear, 3 perpendicular, 1 equal length, 1 midpoint, 1 vertical, 171 other
  measures "d330" radial gap between concentric circles of A11 A37
  measures "d333" radial gap between concentric circles of A32 A46
  measures "d338" radial gap between concentric circles of A3 A51
  measures "d340" radial gap between concentric circles of A31 A53
  measures "d341" radial gap between concentric circles of A19 A54
  measures "d343" radial gap between concentric circles of A14 A56
  measures "d344" radial gap between concentric circles of A33 A57
  measures "d346" radial gap between concentric circles of A5 A59
  measures "d347" radial gap between concentric circles of A20 A60
  measures "d348" radial gap between concentric circles of A23 A61
  measures "d349" distance between parallel lines of L6 L14
  measures "d350" radial gap between concentric circles of A22 A66
  measures "d353" radial gap between concentric circles of A30 A69
  measures "d355" radial gap between concentric circles of A1 A71
  measures "d356" radial gap between concentric circles of A28 A72
  measures "d358" angle of L20 L19
  measures "d359" distance between parallel lines of L19 L29
  measures "d360" distance between parallel lines of L18 L30
  measures "d361" radius of A76
  measures "d362" radius of A79
  measures "d363" distance between parallel lines of L18 L32
  measures "d364" distance between parallel lines of L22 L33
  measures "d365" distance between parallel lines of L21 L34
  measures "d366" distance between parallel lines of L36 L37
  measures "d367" distance between parallel lines of L35 L38
  measures "d368" radius of A85
  measures "d369" radius of A88
  measures "d370" radius of A89
  measures "d371" diameter of A90
  measures "d372" diameter of A91
  measures "d373" diameter of A92
  measures "d374" diameter of A93
  measures "d375" distance between parallel lines of L21 L41
  measures "d376" distance between parallel lines of L39 L42
  measures "d377" distance between parallel lines of L20 L43
  measures "d378" radius of A101
  measures "d379" distance between parallel lines of L20 L44
  measures "d380" distance between parallel lines of L19 L45
  measures "d381" radius of A108
  measures "d382" distance between parallel lines of L39 L46
  measures "d383" distance between parallel lines of L26 L48
  measures "d384" distance between parallel lines of L49 L50
  measures "d385" distance between parallel lines of L51 L52
  measures "d386" distance between parallel lines of L53 L55
  measures "d387" distance between parallel lines of L54 L56
  measures "d388" distance between parallel lines of L35 L57
  measures "d389" radius of A118
  measures "d390" radius of A126
  measures "d391" radius of A131
  measures "d392" diameter of A132
  measures "d393" diameter of A133
body "Solid3"
